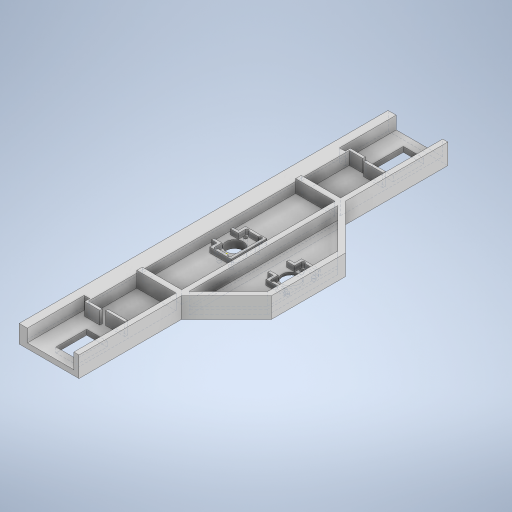
# Autodesk Inventor part: FlanecX_Aax
Saved by Autodesk Inventor 2024 (Build 280153000, 153)
## iProperties
Created: 2023-01-07
Part Number: FlanecX_Aax
Material: Типовые
Document SubType Name: Modeling
Designer: KirikDK
Density: 1 g/cm^3
Appearance: По умолчанию
Mass: 1599.94 g
Surface Area: 2616.33 cm^2
Volume: 1599.94 cm^3
Author: KirikDK
Autodesk Inventor part; units mm, degrees
ref_plane "YZ Plane" through (0, 0, 0) normal (1, 0, 0) x (0, 1, 0)
ref_plane "XZ Plane" through (0, 0, 0) normal (0, 1, 0) x (-1, 0, 0)
ref_plane "XY Plane" through (0, 0, 0) normal (0, 0, 1) x (1, 0, 0)
sketch "Эскиз1" plane through (0, 0, 0) normal (0, 1, 0) x (-1, 0, 0)
  line L0 (45, 341) -> (-42, 341)
  line L1 (-42, 341) -> (-42, -381)
  line L2 (-42, -381) -> (45, -381)
  line L3 (45, -381) -> (45, 341)
  point P0 (0, 0)
  dimension "d0" = 87
  dimension "d1" = 722
  constraints: 8 end point, 2 parallel, 1 horizontal, 1 perpendicular
  measures "d0" distance of L0.start L0.end
  measures "d1" distance of L2.end L0.start
extrude "Выдавливание1" add sketch "Эскиз1" along normal blind 10
sketch "Эскиз2" plane through (0, 10, 0) normal (0, 1, 0) x (1, 0, 0)
  line L0 (26, -320) -> (-14, -320)
  line L1 (-14, -320) -> (-14, -260)
  line L2 (-14, -260) -> (26, -260)
  line L3 (26, -260) -> (26, -320)
  line L4 (-45, -341) -> (42, -341) projected
  line L5 (42, -341) -> (42, 381) projected
  line L6 (42, 381) -> (-45, 381) projected
  line L7 (-319, 20) -> (-306, 20)
  line L8 (26, 360) -> (-14, 360)
  line L9 (-14, 360) -> (-14, 300)
  line L10 (-14, 300) -> (26, 300)
  line L11 (26, 300) -> (26, 360)
  point P0 (0, 0)
  dimension "d4" = 21
  dimension "d5" = 16
  dimension "d6" = 60
  dimension "d7" = 40
  constraints: 18 end point, 4 symmetric about line, 2 horizontal, 2 parallel, 1 perpendicular
  measures "d4" distance between parallel lines of L4 L0
  measures "d5" distance between parallel lines of L5 L3
  measures "d6" distance of L2.end L0.start
  measures "d7" distance of L1.end L2.end
extrude "Выдавливание2" cut sketch "Эскиз2" against normal blind 10
sketch "Эскиз3" plane through (0, 10, 0) normal (0, 1, 0) x (1, 0, 0)
  line L0 (-45, 381) -> (-45, -341) projected
  line L1 (-45, -230) -> (-35, -230)
  line L2 (-35, -230) -> (-35, 270)
  line L3 (-35, 270) -> (-45, 270)
  line L4 (-45, 270) -> (-45, -230)
  line L5 (42, 381) -> (-45, 381) projected
  point P0 (0, 0)
  point P1 (-45, 270)
  dimension "d10" = 10
  dimension "d12" = 500
  dimension "d13" = 111
  constraints: 8 end point, 2 parallel, 1 horizontal, 1 perpendicular, 1 point on line
  measures "d10" distance between parallel lines of L0 L2
  measures "d12" distance of L1.end L2.end
  measures "d13" distance between parallel lines of L5 L3
extrude "Выдавливание3" add sketch "Эскиз3" along normal blind 25
sketch "Эскиз4" plane through (0, 0, 0) normal (0, -1, 0) x (1, 0, 0)
  line L0 (-45, -381) -> (-45, -270) projected
  line L1 (-45, -381) -> (-65, -381)
  line L2 (-65, -381) -> (-65, 341)
  line L3 (-65, 341) -> (-45, 341)
  line L4 (-45, 341) -> (-45, -381)
  line L5 (-45, 341) -> (42, 341) projected
  point P0 (0, 0)
  dimension "d16" = 722
  dimension "d17" = 0
  dimension "d20" = 20
  constraints: 8 end point, 2 parallel, 1 horizontal, 1 perpendicular, 1 point on line
  measures "d16" distance of L1.end L2.end
  measures "d17" distance between parallel lines of L3 L5
  measures "d20" distance of L1.start L1.end
extrude "Выдавливание4" add sketch "Эскиз4" against normal blind 35
sketch "Эскиз6" plane through (0, 0, 0) normal (0, -1, 0) x (1, 0, 0)
  line L0 (-45, 341) -> (42, 341) projected
  line L1 (42, 341) -> (52, 341)
  line L2 (52, 341) -> (52, -381)
  line L3 (52, -381) -> (42, -381)
  line L4 (42, -381) -> (42, 341)
  point P0 (0, 0)
  dimension "d22" = 10
  constraints: 8 end point, 2 parallel, 1 horizontal, 1 perpendicular
  measures "d22" distance of L2.end L3.end
extrude "Выдавливание5" add sketch "Эскиз6" against normal blind 40
sketch "Эскиз7" plane through (0, 10, 0) normal (0, 1, 0) x (1, 0, 0)
  line L0 (-35, -230) -> (-35, 270) projected
  line L1 (42, -341) -> (42, 381) projected
  line L2 (-35, 181) -> (42, 181)
  line L3 (42, 181) -> (42, -141)
  line L4 (42, -141) -> (-35, -141)
  line L5 (-35, -141) -> (-35, 181)
  line L6 (42, 381) -> (-45, 381) projected
  line L7 (-45, -341) -> (42, -341) projected
  line L8 (52, 181) -> (140, 181)
  line L9 (140, 181) -> (140, -141)
  line L10 (140, -141) -> (52, -141)
  line L11 (52, -141) -> (52, 181)
  point P0 (0, 0)
  point P1 (-35, -141)
  point P2 (42, 181)
  dimension "d25" = 200
  dimension "d26" = 200
  constraints: 16 end point, 4 parallel, 2 horizontal, 2 perpendicular, 2 point on line
  measures "d25" distance between parallel lines of L6 L2
  measures "d26" distance between parallel lines of L7 L4
extrude "Выдавливание6" add sketch "Эскиз7" along normal blind 5
sketch "Эскиз8" plane through (0, 15, 0) normal (0, 1, 0) x (1, 0, 0)
  line L0 (-18, 55) -> (24, 55)
  line L1 (24, 55) -> (24, -15)
  line L2 (24, -15) -> (-18, -15)
  line L3 (-18, -15) -> (-18, 55)
  line L4 (42, 381) -> (-45, 381) projected
  line L5 (19, -10) -> (19, 50)
  line L6 (19, 50) -> (-13, 50)
  line L7 (-13, 50) -> (-13, -10)
  line L8 (-13, -10) -> (19, -10)
  line L9 (1, 36) -> (-28.5, 36)
  line L10 (-28.5, 36) -> (-28.5, 4)
  line L11 (-28.5, 4) -> (1, 4)
  line L12 (1, 4) -> (1, 36)
  line L13 (-28.5, 36) -> (-18, 36)
  line L14 (-18, 36) -> (-18, 41)
  line L15 (-18, 41) -> (-28.5, 41)
  line L16 (-28.5, 41) -> (-28.5, 36)
  line L17 (-28.5, 4) -> (-18, 4)
  line L18 (-18, 4) -> (-18, -1)
  line L19 (-18, -1) -> (-28.5, -1)
  line L20 (-28.5, -1) -> (-28.5, 4)
  circle A0 centre (16, 50) radius 3
  circle A1 centre (-10, 50) radius 3
  circle A2 centre (-10, -10) radius 3
  circle A3 centre (16, -10) radius 3
  line L21 (92, 55) -> (134, 55)
  line L22 (134, 55) -> (134, -15)
  line L23 (134, -15) -> (92, -15)
  line L24 (92, -15) -> (92, 55)
  line L25 (129, -10) -> (129, 50)
  line L26 (129, 50) -> (97, 50)
  line L27 (97, 50) -> (97, -10)
  line L28 (97, -10) -> (129, -10)
  line L29 (111, 36) -> (81.5, 36)
  line L30 (81.5, 36) -> (81.5, 4)
  line L31 (81.5, 4) -> (111, 4)
  line L32 (111, 4) -> (111, 36)
  line L33 (81.5, 36) -> (92, 36)
  line L34 (92, 36) -> (92, 41)
  line L35 (92, 41) -> (81.5, 41)
  line L36 (81.5, 41) -> (81.5, 36)
  line L37 (81.5, 4) -> (92, 4)
  line L38 (92, 4) -> (92, -1)
  line L39 (92, -1) -> (81.5, -1)
  line L40 (81.5, -1) -> (81.5, 4)
  circle A4 centre (126, 50) radius 3
  circle A5 centre (100, 50) radius 3
  circle A6 centre (100, -10) radius 3
  circle A7 centre (126, -10) radius 3
  point P0 (0, 0)
  point P1 (-13, 36)
  point P2 (-7, 50)
  point P3 (13, 50)
  point P4 (13, -10)
  point P5 (-7, -10)
  point P6 (-13, 4)
  point P7 (97, 36)
  point P8 (103, 50)
  point P9 (123, 50)
  point P10 (123, -10)
  point P11 (103, -10)
  point P12 (97, 4)
  dimension "d29" = 42
  dimension "d30" = 70
  dimension "d31" = 326
  dimension "d32" = 5
  dimension "d33" = 10.5
  dimension "d47" = 5
  dimension "d48" = 5
  dimension "d49" = 19
  dimension "d50" = 19
  dimension "d61" = 42
  dimension "d62" = 70
  dimension "d63" = 5
  dimension "d64" = 10.5
  dimension "d65" = 5
  dimension "d66" = 5
  dimension "d67" = 19
  dimension "d68" = 19
  constraints: 80 end point, 20 parallel, 12 point on line, 10 perpendicular, 8 horizontal, 30 other
  measures "d29" distance of L0.start L0.end
  measures "d30" distance of L0.end L1.end
  measures "d31" distance between parallel lines of L0 L4
  measures "d32" distance between parallel lines of L1 L5
  measures "d33" distance between parallel lines of L3 L10
  measures "d47" distance between parallel lines of L9 L15
  measures "d48" distance between parallel lines of L19 L11
  measures "d49" distance between parallel lines of L2 L11
  measures "d50" distance between parallel lines of L0 L9
  measures "d61" distance of L21.start L21.end
  measures "d62" distance of L21.end L22.end
  measures "d63" distance between parallel lines of L22 L25
  measures "d64" distance between parallel lines of L24 L30
  measures "d65" distance between parallel lines of L29 L35
  measures "d66" distance between parallel lines of L39 L31
  measures "d67" distance between parallel lines of L23 L31
  measures "d68" distance between parallel lines of L21 L29
extrude "Выдавливание7" add sketch "Эскиз8" along normal blind 10 contours L0 L1 L2 L3 L11 L7 A2 L8 A3 L5 A0 L6 A1 L9 | L3 L9 L16 L15 | L3 L19 L20 L11 | L21 L22 L23 L24 L31 L27 A6 L28 A7 L25 A4 L26 A5 L29 | L24 L29 L36 L35 | L24 L39 L40 L31
sketch "Эскиз9" plane through (0, 15, 0) normal (0, 1, 0) x (1, 0, 0)
  line L0 (-8.75, 45.75) -> (14.75, 45.75)
  line L1 (14.75, 45.75) -> (14.75, -5.75)
  line L2 (14.75, -5.75) -> (-8.75, -5.75)
  line L3 (-8.75, -5.75) -> (-8.75, 45.75)
  line L4 (-28.5, 4) -> (-28.5, -1) projected
  line L5 (-28.5, -1) -> (-18, -1) projected
  line L6 (-18, -1) -> (-18, -15) projected
  line L7 (-18, -15) -> (24, -15) projected
  line L8 (24, -15) -> (24, 55) projected
  line L9 (24, 55) -> (-18, 55) projected
  line L10 (-18, 55) -> (-18, 41) projected
  line L11 (-18, 41) -> (-28.5, 41) projected
  line L12 (-28.5, 41) -> (-28.5, 36) projected
  line L13 (-28.5, 36) -> (-13, 36) projected
  line L14 (-13, 36) -> (-13, 50) projected
  arc A0 (-7, 50) -> (-13, 50) centre (-10, 50) ccw projected
  line L15 (-7, 50) -> (13, 50) projected
  arc A1 (19, 50) -> (13, 50) centre (16, 50) ccw projected
  line L16 (19, 50) -> (19, -10) projected
  arc A2 (13, -10) -> (19, -10) centre (16, -10) ccw projected
  line L17 (13, -10) -> (-7, -10) projected
  arc A3 (-13, -10) -> (-7, -10) centre (-10, -10) ccw projected
  line L18 (-13, -10) -> (-13, 4) projected
  line L19 (-13, 4) -> (-28.5, 4) projected
  circle A4 centre (-8.75, 45.75) radius 3.25
  circle A5 centre (14.75, 45.75) radius 3.25
  circle A6 centre (14.75, -5.75) radius 3.25
  circle A7 centre (-8.75, -5.75) radius 3.25
  circle A8 centre (-4.25, 20) radius 17
  line L20 (101.25, 45.75) -> (124.75, 45.75)
  line L21 (124.75, 45.75) -> (124.75, -5.75)
  line L22 (124.75, -5.75) -> (101.25, -5.75)
  line L23 (101.25, -5.75) -> (101.25, 45.75)
  circle A9 centre (101.25, 45.75) radius 3.25
  circle A10 centre (124.75, 45.75) radius 3.25
  circle A11 centre (124.75, -5.75) radius 3.25
  circle A12 centre (101.25, -5.75) radius 3.25
  circle A13 centre (105.75, 20) radius 17
  point P0 (0, 0)
  dimension "d36" = 4.25
  dimension "d37" = 4.25
  dimension "d38" = 4.25
  dimension "d39" = 4.25
  dimension "d40" = 19
  dimension "d41" = 34
  dimension "d69" = 19
  dimension "d70" = 34
  constraints: 16 end point, 10 centre point, 8 coincident, 4 parallel, 2 horizontal, 2 perpendicular
  measures "d36" distance between parallel lines of L15 L0
  measures "d37" distance between parallel lines of L17 L2
  measures "d38" distance between parallel lines of L16 L1
  measures "d39" distance between parallel lines of L18 L3
  measures "d40" distance from line of L1 A8.centre
  measures "d41" diameter of A8
  measures "d69" distance from line of L21 A13.centre
  measures "d70" diameter of A13
extrude "Выдавливание8" cut sketch "Эскиз9" against normal blind 20 contours L3 A4 L0 | L0 A4 L3 | A5 L1 L0 | L0 L1 A5 | A8 L3 | L3 A8 | A6 L2 L1 | L1 L2 A6 | A7 L2 L3 | L3 L2 A7 | L23 A9 L20 | L20 A9 L23 | A10 L21 L20 | L20 L21 A10 | A13 L23 | L23 A13 | A11 L22 L21 | L21 L22 A11 | A12 L22 L23 | L23 L22 A12
chamfer "Фаска1" [suppressed]
sketch "Эскиз10" plane through (-45, 10, -270) normal (1, 0, 0) x (0, 0, -1)
  line L0 (0, 25) -> (111, 25) projected
  line L1 (0, 0) -> (0, 25) projected
  line L2 (111, 0) -> (0, 0) projected
  line L3 (111, 0) -> (111, 25) projected
  line L4 (-611, 0) -> (-611, 25) projected
  line L5 (-500, 0) -> (-611, 0) projected
  line L6 (-500, 0) -> (-500, 25) projected
  line L7 (-611, 25) -> (-500, 25) projected
  line L8 (111, 0) -> (0, 0) projected
  line L9 (111, 0) -> (111, 25) projected
  line L10 (0, 25) -> (111, 25) projected
  line L11 (0, 0) -> (0, 25) projected
  line L12 (-500, 0) -> (-611, 0) projected
  line L13 (-500, 0) -> (-500, 25) projected
  line L14 (-611, 25) -> (-500, 25) projected
  line L15 (-611, 0) -> (-611, 25) projected
  point P0 (-270, -10)
extrude "Выдавливание9" cut sketch "Эскиз10" against normal blind 2
sketch "Эскиз12" plane through (0, 35, 0) normal (0, 1, 0) x (1, 0, 0)
  line L0 (-35, 270) -> (-45, 270) projected
  line L1 (-38, 270) -> (-8.1221, 270)
  line L2 (-8.1221, 270) -> (-8.1221, 280)
  line L3 (-8.1221, 280) -> (-38, 280)
  line L4 (-38, 280) -> (-38, 270)
  line L5 (35.9063, 275) -> (15.9063, 275)
  line L6 (15.9063, 275) -> (15.9063, 280)
  line L7 (15.9063, 280) -> (35.9063, 280)
  line L8 (35.9063, 280) -> (35.9063, 275)
  circle A0 centre (-4.25, 20) radius 17 projected
  line L9 (-4.25, 20) -> (0, 20)
  line L10 (-35, 269) -> (-35, 274.9994)
  line L11 (-35, 274.9994) -> (10.8519, 274.9994)
  line L12 (35.9063, 275) -> (-1.9378, 275)
  line L13 (-1.9378, 275) -> (-1.9378, 270)
  line L14 (-1.9378, 270) -> (35.9063, 270)
  line L15 (35.9063, 270) -> (35.9063, 275)
  line L16 (-35, -230) -> (-47, -230)
  line L17 (-38, -230) -> (-8.1221, -230)
  line L18 (-8.1221, -230) -> (-8.1221, -240)
  line L19 (-8.1221, -240) -> (-38, -240)
  line L20 (-38, -240) -> (-38, -230)
  line L21 (35.9063, -235) -> (15.9063, -235)
  line L22 (15.9063, -235) -> (15.9063, -240)
  line L23 (15.9063, -240) -> (35.9063, -240)
  line L24 (35.9063, -240) -> (35.9063, -235)
  line L25 (-35, -229) -> (-35, -234.9994)
  line L26 (-35, -234.9994) -> (10.8519, -234.9994)
  line L27 (35.9063, -235) -> (-1.9378, -235)
  line L28 (-1.9378, -235) -> (-1.9378, -230)
  line L29 (-1.9378, -230) -> (35.9063, -230)
  line L30 (35.9063, -230) -> (35.9063, -235)
  point P0 (0, 0)
  point P1 (-47, 270)
  point P2 (-8.1221, -234.9994)
  point P3 (-35, -230)
  point P4 (-8.1221, 274.9994)
  dimension "d56" = 10
  dimension "d57" = 20
  dimension "d58" = 5
  constraints: 60 end point, 16 symmetric about line, 6 parallel, 4 horizontal, 4 perpendicular, 4 point on line, 1 vertical
  measures "d56" distance of L1.end L2.end
  measures "d57" distance of L5.start L5.end
  measures "d58" distance of L5.end L6.end
extrude "Выдавливание11" add sketch "Эскиз12" against normal blind 25 contours L11 L12 L5 L15 L14 L13 | L0 L4 L3 L2 L11 L10 | L25 L26 L18 L19 L20 L16 | L28 L29 L30 L21 L27 L26
sketch "Sketch13" plane through (0, 15, 0) normal (0, 1, 0) x (1, 0, 0)
  point P0 (0, 0)
chamfer "Chamfer2" distance 88 angle 45 2 edges at (140, 12.5, -181) (140, 12.5, 141)
sketch "Sketch14" plane through (0, 0, 0) normal (0, -1, 0) x (1, 0, 0)
  line L0 (52, 141) -> (140, 53)
  line L1 (140, 53) -> (140, -93) projected
  line L2 (140, 53) -> (140, -93)
  line L3 (140, -93) -> (52, -181)
  line L4 (44.2218, 133.2218) -> (129, 48.4437)
  line L5 (129, 48.4437) -> (129, -88.4437)
  line L6 (129, -88.4437) -> (44.2218, -173.2218)
  line L7 (44.2218, -173.2218) -> (52, -181)
  line L8 (44.2218, 133.2218) -> (52, 141)
  line L9 (-35, -181) -> (42, -181) projected
  line L10 (42, -181) -> (-35, -181)
  line L11 (-35, -181) -> (-35, -170)
  line L12 (-35, -170) -> (42, -170)
  line L13 (42, -170) -> (42, -181)
  line L14 (42, 141) -> (-35, 141) projected
  line L15 (42, 141) -> (-35, 141)
  line L16 (-35, 141) -> (-35, 130)
  line L17 (-35, 130) -> (42, 130)
  line L18 (42, 130) -> (42, 141)
  point P0 (0, 0)
  dimension "d75" = 11
  dimension "d78" = 11
  dimension "d79" = 11
  constraints: 32 end point, 5 equal length, 5 perpendicular, 2 horizontal, 1 point on line, 2 other
  measures "d75" distance between parallel lines of L5 L1
  measures "d78" distance of L15.end L16.end
  measures "d79" distance of L10.end L11.end
extrude "Extrusion12" add sketch "Sketch14" against normal blind 40
sketch "Sketch15" plane through (-47, 10, -270) normal (1, 0, 0) x (0, 0, -1)
  line L0 (111, 25) -> (111, 0) projected
  line L1 (111, 25) -> (0, 25)
  line L2 (0, 25) -> (0, 0)
  line L3 (0, 0) -> (111, 0)
  line L4 (111, 0) -> (111, 25)
  line L5 (-500, 0) -> (-500, 25) projected
  line L6 (-611, 25) -> (-500, 25)
  line L7 (-500, 25) -> (-500, 0)
  line L8 (-500, 0) -> (-611, 0)
  line L9 (-611, 0) -> (-611, 25)
  point P0 (-270, -10)
  point P1 (111, 0)
  constraints: 16 end point, 4 parallel, 2 horizontal, 2 perpendicular
extrude "Extrusion13" cut sketch "Sketch15" against normal blind 2
